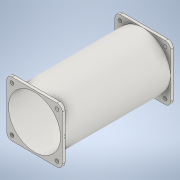
# Autodesk Inventor part: Gehäuse
Saved by Autodesk Inventor 2020.3 (Build 243373000, 373)
## iProperties
Created: 2021-05-14
Part Number: Gehäuse
Material: Stahl AISI 1080
Document SubType Name: Modeling
Designer: user
Density: 7.85 g/cm^3
Appearance: Stahl
Author: user
Autodesk Inventor part; units mm, degrees
ref_plane "YZ Plane" through (0, 0, 0) normal (1, 0, 0) x (0, 1, 0)
ref_plane "XZ Plane" through (0, 0, 0) normal (0, 1, 0) x (-1, 0, 0)
ref_plane "XY Plane" through (0, 0, 0) normal (0, 0, 1) x (1, 0, 0)
sketch "Skizze1" plane through (0, 0, 0) normal (0, 1, 0) x (-1, 0, 0)
  line L0 (0, 0) -> (80, 0)
  line L1 (80, 0) -> (80, -152)
  line L2 (80, -152) -> (0, -152)
  line L3 (0, -152) -> (0, 0)
  line L4 (80, -152) -> (-80, -152)
  line L5 (-80, -152) -> (-80, -160)
  line L6 (-80, -160) -> (80, -160)
  line L7 (80, -160) -> (80, -152)
  dimension "d0" = 160
  dimension "d1" = 160
  dimension "d2" = 8
  constraints: 16 end point, 4 parallel, 2 horizontal, 2 perpendicular, 1 midpoint, 1 point on line
  measures "d0" diameter of L1 L3
  measures "d1" distance between parallel lines of L6 L0
  measures "d2" distance of L4.end L5.end
revolve "Umdrehung1" add sketch "Skizze1" angle 360 about axis through (0, 0, -152) along (0, 0, 1) contours L0 L1 L2 L3
extrude "Extrusion1" add sketch "Skizze1" along normal mid plane 160 contours L2 L7 L6 L5 L4
fillet "Rundung1" radius 15 4 edges at (80, 80, -156) (-80, 80, -156) (80, -80, -156) (-80, -80, -156)
sketch "Skizze2" plane through (65, 80, -160) normal (0, 0, -1) x (-1, 0, 0)
  circle A0 centre (65, -80) radius 80 projected
  constraints: 1 coincident
hole "Bohrung1" at (0, 0, -160) direction (0, 0, 1) diameter 150 end through all
sketch "Skizze3" plane through (65, 80, -160) normal (0, 0, -1) x (-1, 0, 0)
  line L0 (130, -145) -> (0, -145)
  line L1 (0, -145) -> (0, -15)
  line L2 (0, -15) -> (130, -15)
  line L3 (130, -15) -> (130, -145)
  line L4 (130, -145) -> (0, -15) construction
  line L5 (0, -145) -> (130, -15) construction
  point P0 (65, -80)
  dimension "d14" = 130
  dimension "d15" = 130
  constraints: 12 end point, 2 midpoint, 2 parallel, 1 horizontal, 1 perpendicular
  measures "d14" distance of L1.end L2.end
  measures "d15" distance of L0.end L1.end
hole "Bohrung2" at (-65, 65, -160) at (65, 65, -160) at (65, -65, -160) at (-65, -65, -160) direction (0, 0, 1) diameter 10.5 end through all
mirror "Spiegeln1" about plane through (-80, 0, 0) normal (0, 0, 1)
equation "\"d4\" = d0"
